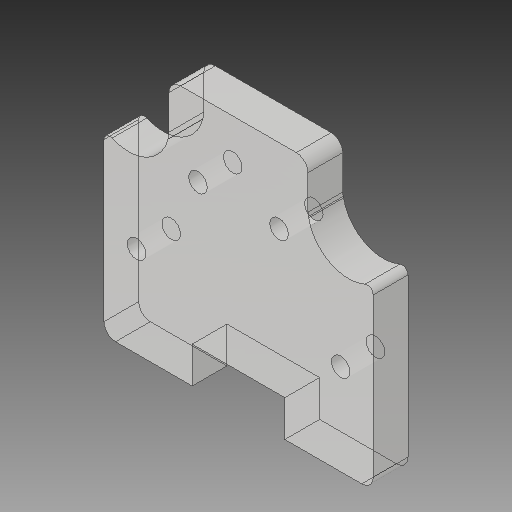
# Autodesk Inventor part: Hotend Slide Part3
Saved by Autodesk Inventor 2018 (Build 220112000, 112)
## iProperties
Created: 2016-06-24
Part Number: Hotend Slide Part3
Material: PET Plastic
Document SubType Name: Modeling
Designer: joshm
Density: 1.541 g/cm^3
Appearance: Polycarbonate - Clear
Mass: 14.8455 g
Surface Area: 45.6025 cm^2
Volume: 9.63365 cm^3
Author: joshm
Autodesk Inventor part; units mm, degrees
ref_plane "YZ Plane" through (0, 0, 0) normal (1, 0, 0) x (0, 1, 0)
ref_plane "XZ Plane" through (0, 0, 0) normal (0, 1, 0) x (-1, 0, 0)
sketch "Sketch1" plane through (0, 0, 0) normal (0, 0, 1) x (1, 0, 0)
  line L0 (-23.2294, -5.2752) -> (-23.2294, 25.7248)
  arc A0 (-23.2294, 25.7248) -> (-11.9794, 30.7248) centre (-18.9581, 31.2706) ccw
  line L1 (0.0206, 30.7248) -> (-11.9794, 30.7248)
  line L2 (0.0206, 30.7248) -> (12.0206, 30.7248)
  arc A1 (12.0206, 30.7248) -> (23.2706, 25.7248) centre (18.9993, 31.2706) ccw
  line L3 (23.2706, -5.2752) -> (23.2706, 25.7248)
  circle A2 centre (17.6456, 10.4258) radius 1.6
  circle A3 centre (-17.6044, 10.4258) radius 1.6
  line L4 (-23.2294, -5.2752) -> (23.2706, -5.2752)
  point P0 (0, 0)
  point P1 (0, -3.0755)
  constraints: 10 end point, 4 centre point, 4 point on circle, 1 horizontal
extrude "Extrusion1" add sketch "Sketch1" along normal blind 6
sketch "Sketch2" plane through (0, 0, 6) normal (0, 0, 1) x (1, 0, 0)
  circle A0 centre (-6.9972, 25.6961) radius 1.6 projected
  circle A1 centre (7.0028, 25.7124) radius 1.6 projected
  point P0 (0, 0)
extrude "Extrusion2" cut sketch "Sketch2" against normal through all
fillet "Fillet1" radius 1 4 edges at (-11.9794, 30.7248, 3) (-23.2294, 25.7248, 3) (12.0206, 30.7248, 3) (23.2706, 25.7248, 3)
fillet "Fillet2" radius 2 2 edges at (-23.2294, -5.2752, 3) (23.2706, -5.2752, 3)
sketch "Sketch3" plane through (0, 0, 6) normal (0, 0, 1) x (1, 0, 0)
  line L0 (0, 0.9807) -> (-8, 0.9807)
  line L1 (0, 0.9807) -> (8, 0.9807) construction
  line L2 (-8, 0.9807) -> (8, 0.9807)
  line L3 (8, 0.9807) -> (8, -5.2752)
  line L4 (21.2706, -5.2752) -> (-21.2294, -5.2752) projected
  line L5 (-8, 0.9807) -> (-8, -5.2752)
  point P0 (0, 0)
  dimension "d6" = 8
  dimension "d7" = 180
  dimension "d8" = 16
  dimension "d9" = 0
  constraints: 10 end point, 2 collinear, 2 horizontal, 2 point on line, 1 parallel, 1 perpendicular
  measures "d6" distance of L0.start L0.end
  measures "d7" angle of L0 L1
  measures "d8" distance of L0.end L2.end
  measures "d9" distance between parallel lines of L2 L0
extrude "Extrusion3" cut sketch "Sketch3" against normal blind 10
sketch "Sketch4" plane through (0, 0, 6) normal (0, 0, 1) x (1, 0, 0)
  arc A0 (6.0143, -33.637) -> (7.9856, -35.2865) centre (7.9833, -33.2865) ccw projected
  line L0 (7.9856, -35.2865) -> (21.3237, -35.271) projected
  arc A1 (21.3237, -35.271) -> (23.3214, -33.2687) centre (21.3214, -33.271) ccw projected
  line L1 (23.3214, -33.2687) -> (23.2549, 23.9765) projected
  arc A2 (23.2549, 23.9765) -> (21.8449, 24.8874) centre (22.2549, 23.9753) ccw projected
  arc A3 (11.997, 30.7182) -> (21.8449, 24.8874) centre (18.9751, 31.2721) ccw projected
  line L2 (11.997, 30.7182) -> (11.9902, 36.6182) projected
  arc A4 (11.9902, 36.6182) -> (9.9879, 38.6159) centre (9.9902, 36.6159) ccw projected
  line L3 (9.9879, 38.6159) -> (2.4879, 38.6072) projected
  arc A5 (2.4879, 38.6072) -> (1.489, 37.606) centre (2.489, 37.6072) ccw projected
  line L4 (1.489, 37.606) -> (1.4937, 33.606) projected
  line L5 (1.4937, 33.606) -> (2.7437, 33.6075) projected
  line L6 (2.7437, 33.6075) -> (2.747, 30.7075) projected
  line L7 (2.747, 30.7075) -> (1.547, 30.7061) projected
  line L8 (1.547, 30.7061) -> (1.5587, 20.7061) projected
  line L9 (1.5587, 20.7061) -> (10.0087, 20.7159) projected
  arc A6 (12.011, 18.7182) -> (10.0087, 20.7159) centre (10.011, 18.7159) ccw projected
  line L10 (12.011, 18.7182) -> (12.0365, -3.2818) projected
  arc A7 (12.0365, -3.2818) -> (14.0389, -5.2794) centre (14.0365, -3.2794) ccw projected
  line L11 (14.0389, -5.2794) -> (16.2889, -5.2768) projected
  arc A8 (18.2912, -7.2745) -> (16.2889, -5.2768) centre (16.2912, -7.2768) ccw projected
  line L12 (18.2912, -7.2745) -> (18.3109, -24.2745) projected
  arc A9 (16.3133, -26.2768) -> (18.3109, -24.2745) centre (16.3109, -24.2768) ccw projected
  line L13 (16.3133, -26.2768) -> (-16.1867, -26.3146) projected
  arc A10 (-18.189, -24.3169) -> (-16.1867, -26.3146) centre (-16.189, -24.3146) ccw projected
  line L14 (-18.189, -24.3169) -> (-18.2088, -7.3169) projected
  arc A11 (-16.2111, -5.3146) -> (-18.2088, -7.3169) centre (-16.2088, -7.3146) ccw projected
  line L15 (-16.2111, -5.3146) -> (-13.9611, -5.312) projected
  arc A12 (-13.9611, -5.312) -> (-11.9634, -3.3096) centre (-13.9634, -3.312) ccw projected
  line L16 (-11.9634, -3.3096) -> (-11.989, 18.6903) projected
  arc A13 (-9.9913, 20.6927) -> (-11.989, 18.6903) centre (-9.989, 18.6927) ccw projected
  line L17 (-9.9913, 20.6927) -> (-1.5413, 20.7025) projected
  line L18 (-1.5413, 20.7025) -> (-1.553, 30.7025) projected
  line L19 (-1.553, 30.7025) -> (-2.753, 30.7011) projected
  line L20 (-2.753, 30.7011) -> (-2.7563, 33.6011) projected
  line L21 (-2.7563, 33.6011) -> (-1.5063, 33.6025) projected
  line L22 (-1.5063, 33.6025) -> (-1.511, 37.6025) projected
  arc A14 (-1.511, 37.6025) -> (-2.5121, 38.6014) centre (-2.511, 37.6014) ccw projected
  line L23 (-2.5121, 38.6014) -> (-10.0121, 38.5926) projected
  arc A15 (-10.0121, 38.5926) -> (-12.0098, 36.5903) centre (-10.0098, 36.5926) ccw projected
  line L24 (-12.0098, 36.5903) -> (-12.0029, 30.6903) projected
  arc A16 (-21.8372, 24.8367) -> (-12.0029, 30.6903) centre (-18.9823, 31.228) ccw projected
  arc A17 (-21.8372, 24.8367) -> (-23.2451, 23.9225) centre (-22.2451, 23.9236) ccw projected
  line L25 (-23.2451, 23.9225) -> (-23.1786, -33.3227) projected
  arc A18 (-23.1786, -33.3227) -> (-21.1762, -35.3204) centre (-21.1786, -33.3204) ccw projected
  line L26 (-21.1762, -35.3204) -> (-7.8381, -35.3049) projected
  arc A19 (-7.8381, -35.3049) -> (-5.8706, -33.6509) centre (-7.8405, -33.3049) ccw projected
  arc A20 (6.0143, -33.637) -> (-5.8706, -33.6509) centre (0.073, -34.6948) ccw projected
  circle A21 centre (17.6456, 10.4258) radius 1.6 projected
  circle A22 centre (-17.6044, 10.3848) radius 1.6 projected
  circle A23 centre (7.0029, 25.7124) radius 1.6 projected
  circle A24 centre (-6.9971, 25.6961) radius 1.6 projected
  line L27 (11.1501, 30.7248) -> (-11.1088, 30.7248) projected
  line L28 (-2.5121, 38.6014) -> (2.4879, 38.6072)
  line L29 (-12.1907, 29.5326) -> (12.1947, 29.5326)
  point P0 (0, 0)
  constraints: 4 end point, 2 point on circle, 1 collinear, 1 horizontal, 1 tangent
ref_plane "Work Plane1" through (-23.2654, -35.3247, 0) normal (0, 0, 1) x (1, 0.0012, 0)
extrude "Extrusion4" add sketch "Sketch4" against normal up to surface (6 mm away) contours L29 L8 L7 L6 L5 L4 A5 L3 A4 L2 A3 | L29 L18 L19 L20 L27 L6 L7 L8 | A16 L24 A15 L23 A14 L22 L21 L20 L19 L18 L29 | A5 L4 L5 L6 L27 L20 L21 L22 A14 L28
body "Solid1"
